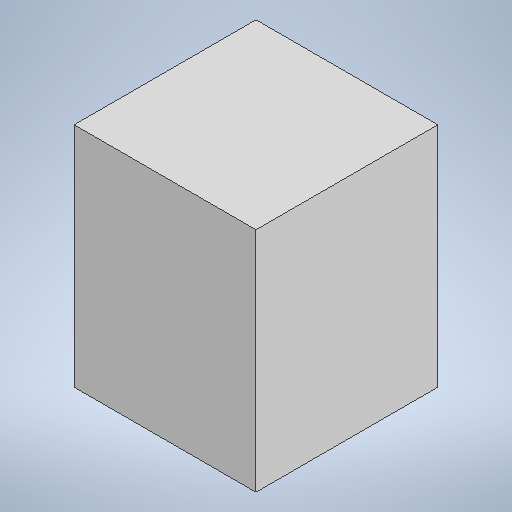
# Autodesk Inventor part: Stützblöcke
Saved by Autodesk Inventor 2025.2 (Build 292293000, 293)
## iProperties
Created: 2024-11-13
Part Number: Stützblöcke
Material: Generisch
Document SubType Name: Modeling
Designer: tills
Density: 1 g/cm^3
Appearance: Vorgabe
Author: tills
Autodesk Inventor part; units mm, degrees
ref_plane "YZ Plane" through (0, 0, 0) normal (1, 0, 0) x (0, 1, 0)
ref_plane "XZ Plane" through (0, 0, 0) normal (0, 1, 0) x (-1, 0, 0)
ref_plane "XY Plane" through (0, 0, 0) normal (0, 0, 1) x (1, 0, 0)
sketch "Skizze1" plane through (0, 0, 0) normal (0, 1, 0) x (-1, 0, 0)
  line L0 (-20, 20) -> (20, 20)
  line L1 (20, 20) -> (20, -20)
  line L2 (20, -20) -> (-20, -20)
  line L3 (-20, -20) -> (-20, 20)
  line L4 (-20, 20) -> (20, -20) construction
  line L5 (20, 20) -> (-20, -20) construction
  line L6 (20, 20) -> (0, 20) construction
  line L7 (0, 20) -> (0, 0) construction
  line L8 (0, 0) -> (20, 0) construction
  line L9 (20, 0) -> (20, 20) construction
  line L10 (0, 0) -> (-20, 0) construction
  line L11 (-20, 0) -> (-20, -20) construction
  line L12 (-20, -20) -> (0, -20) construction
  line L13 (0, -20) -> (0, 0) construction
  point P0 (10, 10)
  point P1 (-10, -10)
  dimension "d0" = 40
  dimension "d1" = 40
  constraints: 28 end point, 6 parallel, 3 horizontal, 3 perpendicular, 2 midpoint, 2 point on line
  measures "d0" distance of L0.end L1.end
  measures "d1" distance of L1.end L2.end
extrude "Extrusion1" add sketch "Skizze1" along normal blind 10
sketch "Skizze2" plane through (0, 0, 0) normal (0, -1, 0) x (1, 0, 0)
  line L0 (20, -20) -> (-20, -20) construction
  line L1 (20, 20) -> (20, -20) construction
  line L2 (-20, 20) -> (20, 20) construction
  line L3 (-20, -20) -> (-20, 20) construction
  line L4 (20, 20) -> (0, 20) construction
  line L5 (0, 20) -> (0, 0) construction
  line L6 (0, 0) -> (20, 0) construction
  line L7 (20, 0) -> (20, 20) construction
  line L8 (-20, -20) -> (0, -20) construction
  line L9 (0, -20) -> (0, 0) construction
  line L10 (0, 0) -> (-20, 0) construction
  line L11 (-20, 0) -> (-20, -20) construction
  circle A0 centre (10, 10) radius 5
  circle A1 centre (-10, -10) radius 5
  dimension "d4" = 10
  dimension "d5" = 10
  constraints: 16 end point, 4 parallel, 2 centre point, 2 coincident, 2 horizontal, 2 perpendicular
  measures "d4" diameter of A0
  measures "d5" diameter of A1
extrude "Extrusion2" cut sketch "Skizze2" against normal blind 5
sketch "Skizze4" plane through (0, 0, 0) normal (0, -1, 0) x (1, 0, 0)
  line L0 (20, 20) -> (20, -20) projected
  line L1 (-20, -20) -> (-20, 20) projected
  line L2 (-20, 20) -> (20, 20) projected
  line L3 (20, -20) -> (-20, -20) projected
  line L4 (20, 20) -> (-20, 20)
  line L5 (-20, 20) -> (-20, -20)
  line L6 (-20, -20) -> (20, -20)
  line L7 (20, -20) -> (20, 20)
  point P0 (0, 0)
  constraints: 8 end point, 2 parallel, 1 horizontal, 1 perpendicular
extrude "Extrusion3" add sketch "Skizze4" along normal blind 40
sketch "Skizze5" plane through (0, -40, 0) normal (0, -1, 0) x (1, 0, 0)
  line L0 (20, -20) -> (20, 20) projected
  line L1 (20, 20) -> (-20, 20) projected
  line L2 (-20, 20) -> (-20, -20) projected
  line L3 (-20, -20) -> (20, -20) projected
  line L4 (-20, 20) -> (0, 20) construction
  line L5 (0, 20) -> (0, 0) construction
  line L6 (0, 0) -> (-20, 0) construction
  line L7 (-20, 0) -> (-20, 20) construction
  line L8 (0, -20) -> (20, -20) construction
  line L9 (20, -20) -> (20, 0) construction
  line L10 (20, 0) -> (0, 0) construction
  line L11 (0, 0) -> (0, -20) construction
  circle A0 centre (-10, 10) radius 2.5
  circle A1 centre (10, -10) radius 2.5
  dimension "d10" = 5
  dimension "d11" = 5
  constraints: 16 end point, 4 parallel, 2 centre point, 2 coincident, 2 horizontal, 2 midpoint, 2 perpendicular
  measures "d10" diameter of A1
  measures "d11" diameter of A0
hole "Bohrung1" at (-10, -40, 10) at (10, -40, -10) direction (0, 1, 0) diameter 5 depth 10
